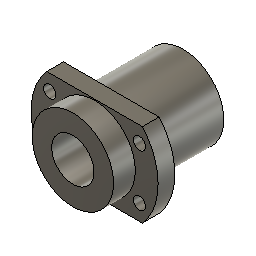
Prototype_1_reducer v30 (Autodesk Fusion 360 archive; units mm, degrees)
design "SFY4040-3.6"
Autodesk Fusion 360 part; units mm, degrees
sketch "Sketch1" plane through (0, 0, 0) normal (0, 0, 1) x (1, 0, 0)
  circle A0 centre (0, 0) radius 19
  circle A1 centre (0, 0) radius 57
  circle A2 centre (0, 0) radius 46.5 construction
  line L0 (57, 37.5) -> (-57, 37.5)
  line L1 (-57, 37.5) -> (-57, -37.5)
  line L2 (-57, -37.5) -> (57, -37.5)
  line L3 (57, -37.5) -> (57, 37.5)
  line L4 (57, 37.5) -> (-57, -37.5) construction
  line L5 (-57, 37.5) -> (57, -37.5) construction
  circle A3 centre (0, 0) radius 36.5
  dimension "d1" = 38
  dimension "d2" = 114
  dimension "d3" = 93
  dimension "d4" = 75
  dimension "d5" = 114
  dimension "d6" = 73
  constraint coincident A0.centre A1.centre
  constraint concentric A1 A2
  constraint perpendicular L0 L1
  constraint parallel L0 L2
  constraint parallel L1 L3
  constraint horizontal L0
  constraint coincident L4 A0.centre
  constraint coincident L5 A0.centre
  constraint concentric A2 A3
  measures "d1" diameter of A0
  measures "d2" diameter of A1
  measures "d3" diameter of A2
  measures "d4" distance of L0.start L2.end
  measures "d5" distance of L0.start L0.end
  measures "d6" diameter of A3
extrude "Extrude1" add sketch "Sketch1" against normal blind 15 contours A1 L0 L2 | A3
extrude "Extrude2" add sketch "Sketch1" along normal blind 19.5 contours A3
sketch "Sketch2" plane through (0, 0, -15) normal (0, 0, -1) x (-1, 0, 0)
  circle A0 centre (0, 0) radius 19
  arc A1 (42.9273, -37.5) -> (42.9273, 37.5) centre (0, 0) ccw
  line L0 (42.9273, 37.5) -> (-42.9273, 37.5)
  arc A2 (-42.9273, 37.5) -> (-42.9273, -37.5) centre (0, 0) ccw
  line L1 (-42.9273, -37.5) -> (42.9273, -37.5)
  circle A3 centre (0, 0) radius 36.5
  circle A4 centre (0, 0) radius 36.5
extrude "Extrude3" add sketch "Sketch2" along normal blind 64.5 contours A3 A4
sketch "Sketch3" plane through (0, 0, 0) normal (0, 0, 1) x (1, 0, 0)
  circle A0 centre (0, 0) radius 36.5
  arc A1 (-42.9273, 37.5) -> (-42.9273, -37.5) centre (0, 0) ccw
  line L0 (-42.9273, -37.5) -> (42.9273, -37.5)
  arc A2 (42.9273, -37.5) -> (42.9273, 37.5) centre (0, 0) ccw
  line L1 (42.9273, 37.5) -> (-42.9273, 37.5)
  circle A3 centre (0, 0) radius 46.5 construction
  line L2 (-57, -37.5) -> (57, -37.5)
  line L3 (57, -37.5) -> (57, 37.5)
  line L4 (-57, 37.5) -> (-57, -37.5)
  line L5 (57, 37.5) -> (-57, 37.5)
  line L6 (0, 0) -> (57, 0) construction
  circle A4 centre (40.2702, 23.25) radius 5.5
  line L7 (0, 0) -> (40.2702, 23.25)
  line L8 (0, 0) -> (0, 36.5) construction
  circle A5 centre (40.2702, -23.25) radius 5.5
  circle A6 centre (-40.2702, -23.25) radius 5.5
  circle A7 centre (-40.2702, 23.25) radius 5.5
  dimension "d13" = 11
  dimension "d14" = 30
  constraint coincident A0.centre A1.centre
  constraint midpoint L3 L6.end
  constraint coincident A3 A4.centre
  constraint coincident A4.centre L7.end
  constraint coincident A0 L8.end
  constraint perpendicular L6 L8
  constraint symmetric L6 A4 A5
  constraint symmetric A4 L8 A7
  constraint symmetric L8 A5 A6
  measures "d13" diameter of A4
  measures "d14" angle of L6 L7
extrude "Extrude4" cut sketch "Sketch3" against normal blind 16.266 contours A4 | A5 | A6 | A7

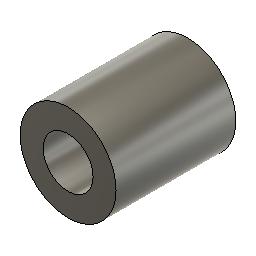
design "RCL48-2525"
Autodesk Fusion 360 part; units mm, degrees
sketch "Sketch1" plane through (0, 0, 0) normal (0, 0, 1) x (1, 0, 0)
  circle A0 centre (0, 0) radius 24
  dimension "d1" = 48
  constraint coincident A0.centre origin
  measures "d1" diameter of A0
extrude "Extrude1" add sketch "Sketch1" against normal blind 60
sketch "Sketch2" plane through (0, 0, 0) normal (0, 0, 1) x (1, 0, 0)
  circle A0 centre (0, 0) radius 24
  circle A1 centre (0, 0) radius 12.5
  dimension "d4" = 25
  constraint concentric A0 A1
  measures "d4" diameter of A1
extrude "Extrude2" cut sketch "Sketch2" against normal blind 84.022 contours A1

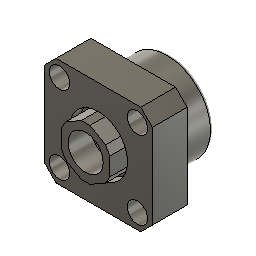
design "FK30"
Autodesk Fusion 360 part; units mm, degrees
sketch "Sketch1" plane through (0, 0, 0) normal (0, 0, 1) x (1, 0, 0)
  line L0 (46.5, 46.5) -> (-46.5, 46.5)
  line L1 (-46.5, 46.5) -> (-46.5, -46.5)
  line L2 (-46.5, -46.5) -> (46.5, -46.5)
  line L3 (46.5, -46.5) -> (46.5, 46.5)
  line L4 (46.5, 46.5) -> (-46.5, -46.5) construction
  line L5 (-46.5, 46.5) -> (46.5, -46.5) construction
  dimension "d1" = 93
  dimension "d2" = 93
  constraint perpendicular L0 L1
  constraint parallel L0 L2
  constraint parallel L1 L3
  constraint horizontal L0
  constraint coincident L4 origin
  constraint coincident L5 origin
  measures "d1" distance of L0.start L0.end
  measures "d2" distance of L0.start L2.end
extrude "Extrude1" add sketch "Sketch1" against normal blind 30 makes body 1
sketch "Sketch2" plane through (0, 0, -30) normal (0, 0, -1) x (-1, 0, 0)
  line L0 (-46.5, 46.5) -> (-46.5, -46.5)
  line L1 (-46.5, -46.5) -> (46.5, -46.5)
  line L2 (46.5, -46.5) -> (46.5, 46.5)
  line L3 (46.5, 46.5) -> (-46.5, 46.5)
  circle A0 centre (0, 0) radius 37.5
  dimension "d5" = 75
  constraint coincident A0.centre origin
  measures "d5" diameter of A0
extrude "Extrude2" add sketch "Sketch2" along normal blind 32 contours A0 bodies 1
sketch "Sketch3" plane through (0, 0, 0) normal (0, 0, 1) x (1, 0, 0)
  line L0 (46.5, -46.5) -> (46.5, 46.5)
  line L1 (46.5, 46.5) -> (-46.5, 46.5)
  line L2 (-46.5, 46.5) -> (-46.5, -46.5)
  line L3 (-46.5, -46.5) -> (46.5, -46.5)
  circle A0 centre (0, 0) radius 47.5 construction
  circle A1 centre (33.5876, 33.5876) radius 5.5
  circle A2 centre (33.5876, -33.5876) radius 5.5
  circle A3 centre (-33.5876, -33.5876) radius 5.5
  circle A4 centre (-33.5876, 33.5876) radius 5.5
  line L4 (0, 0) -> (46.5, 0) construction
  line L5 (33.5876, 33.5876) -> (0, 0) construction
  dimension "d8" = 95
  dimension "d9" = 11
  dimension "d10" = 45
  constraint coincident A0.centre L4.start
  constraint coincident A0 A1.centre
  constraint coincident A0 A2.centre
  constraint coincident A0 A3.centre
  constraint coincident A0 A4.centre
  constraint equal A1 A4
  constraint equal A3 A4
  constraint equal A2 A3
  constraint midpoint L0 L4.end
  constraint coincident A1.centre L5.start
  constraint horizontal A4.centre A1.centre
  constraint vertical A3.centre A4.centre
  constraint horizontal A2.centre A3.centre
  measures "d8" diameter of A0
  measures "d9" diameter of A1
  measures "d10" angle of L4 L5
extrude "Extrude3" cut sketch "Sketch3" against normal blind 34.907 contours A1 | A2 | A3 | A4 bodies 1
sketch "Sketch4" plane through (0, 0, 0) normal (0, 0, 1) x (1, 0, 0)
  circle A0 centre (-33.5876, 33.5876) radius 5.5
  circle A1 centre (-33.5876, -33.5876) radius 5.5
  circle A2 centre (33.5876, 33.5876) radius 5.5
  circle A3 centre (33.5876, -33.5876) radius 5.5
  line L0 (46.5, -46.5) -> (46.5, 46.5)
  line L1 (46.5, 46.5) -> (-46.5, 46.5)
  line L2 (-46.5, 46.5) -> (-46.5, -46.5)
  line L3 (-46.5, -46.5) -> (46.5, -46.5)
  circle A4 centre (33.5876, 33.5876) radius 8.75
  circle A5 centre (-33.5876, 33.5876) radius 8.75
  circle A6 centre (-33.5876, -33.5876) radius 8.75
  circle A7 centre (33.5876, -33.5876) radius 8.75
  dimension "d13" = 17.5
  constraint concentric A2 A4
  constraint concentric A0 A5
  constraint concentric A1 A6
  constraint concentric A3 A7
  constraint equal A4 A5
  constraint equal A5 A6
  constraint equal A6 A7
  measures "d13" diameter of A4
extrude "Extrude4" cut sketch "Sketch4" against normal blind 15 contours A4 | A5 | A6 | A7 bodies 1
sketch "Sketch5" plane through (0, 0, 0) normal (0, 0, 1) x (1, 0, 0)
  circle A0 centre (-33.5876, 33.5876) radius 8.75
  circle A1 centre (-33.5876, -33.5876) radius 8.75
  circle A2 centre (33.5876, 33.5876) radius 8.75
  circle A3 centre (33.5876, -33.5876) radius 8.75
  line L0 (46.5, -46.5) -> (46.5, 46.5)
  line L1 (46.5, 46.5) -> (-46.5, 46.5)
  line L2 (-46.5, 46.5) -> (-46.5, -46.5)
  line L3 (-46.5, -46.5) -> (46.5, -46.5)
  circle A4 centre (0, 0) radius 15
  dimension "d16" = 30
  constraint coincident A4.centre origin
  measures "d16" diameter of A4
extrude "Extrude5" cut sketch "Sketch5" against normal blind 68.719 contours A4 bodies 1
sketch "Sketch6" plane through (0, 0, 0) normal (0, 0, 1) x (1, 0, 0)
  circle A0 centre (0, 0) radius 15
  circle A1 centre (-33.5876, 33.5876) radius 8.75
  circle A2 centre (-33.5876, -33.5876) radius 8.75
  circle A3 centre (33.5876, 33.5876) radius 8.75
  circle A4 centre (33.5876, -33.5876) radius 8.75
  line L0 (46.5, -46.5) -> (46.5, 46.5)
  line L1 (46.5, 46.5) -> (-46.5, 46.5)
  line L2 (-46.5, 46.5) -> (-46.5, -46.5)
  line L3 (-46.5, -46.5) -> (46.5, -46.5)
  circle A5 centre (0, 0) radius 25
  dimension "d19" = 50
  constraint concentric A0 A5
  measures "d19" diameter of A5
extrude "Extrude6" cut sketch "Sketch6" against normal blind 9 contours A5 bodies 1
sketch "Sketch7" plane through (0, 0, -9) normal (0, 0, 1) x (1, 0, 0)
  circle A0 centre (0, 0) radius 15
  circle A1 centre (0, 0) radius 25
  circle A2 centre (0, 0) radius 22.5
  dimension "d22" = 45
  constraint concentric A0 A2
  measures "d22" diameter of A2
extrude "Extrude7" cut sketch "Sketch7" against normal blind 9 contours A2 bodies 1
sketch "Sketch8" plane through (0, 0, -18) normal (0, 0, 1) x (1, 0, 0)
  circle A0 centre (0, 0) radius 15
  circle A1 centre (0, 0) radius 22.5
  circle A2 centre (0, 0) radius 17.4
  dimension "d25" = 34.8
  constraint concentric A0 A2
  measures "d25" diameter of A2
extrude "Extrude8" add sketch "Sketch8" along normal blind 9 separate body contours A2 makes body 2
sketch "Sketch9" plane through (0, 0, -62) normal (0, 0, -1) x (-1, 0, 0)
  circle A0 centre (0, 0) radius 15
  circle A1 centre (0, 0) radius 37.5
  circle A2 centre (0, 0) radius 22.5
  dimension "d28" = 45
  constraint concentric A0 A2
  measures "d28" diameter of A2
extrude "Extrude9" cut sketch "Sketch9" against normal blind 12 contours A2 bodies 1
sketch "Sketch10" plane through (0, 0, -50) normal (0, 0, -1) x (-1, 0, 0)
  circle A0 centre (0, 0) radius 15
  circle A1 centre (0, 0) radius 22.5
  circle A2 centre (0, 0) radius 17.4
  dimension "d31" = 34.8
  constraint coincident A0.centre A1.centre
  measures "d31" diameter of A2
extrude "Extrude10" add sketch "Sketch10" along normal blind 9 separate body contours A2 makes body 3
chamfer "Chamfer1" distance 10 angle 45 4 edges at (46.5, 46.5, -15) (-46.5, 46.5, -15) (46.5, -46.5, -15) (-46.5, -46.5, -15) on bodies 1
fillet "Fillet1" radius 3 1 edges at (34.9623, -13.5606, -62) on bodies 1
sketch "Sketch11" plane through (0, 0, -9) normal (0, 0, 1) x (1, 0, 0)
  circle A0 centre (0, 0) radius 15
  circle A1 centre (0, 0) radius 17.4
  line L0 (0, 31.1127) -> (0, -31.1127) construction
  line L1 (-12.7017, 22) -> (-25.4034, 0)
  line L2 (-25.4034, 0) -> (-12.7017, -22)
  line L3 (-12.7017, -22) -> (12.7017, -22)
  line L4 (12.7017, -22) -> (25.4034, 0)
  line L5 (25.4034, 0) -> (12.7017, 22)
  line L6 (12.7017, 22) -> (-12.7017, 22)
  dimension "d43" = 22
  constraint coincident A0.centre A1.centre
  constraint coincident L0 A0.centre
  constraint vertical L0
  constraint horizontal L6
  measures "d43" distance of A0.centre L6
extrude "Extrude11" add sketch "Sketch11" along normal blind 20 separate body contours A1 | L1 L2 L3 L4 L5 L6 makes body 4
chamfer "Chamfer4" distance 9 angle 45 6 edges at (12.7017, 22, 1) (25.4034, 0, 1) (12.7017, -22, 1) (-12.7017, -22, 1) (-25.4034, 0, 1) (-12.7017, 22, 1) on bodies 4

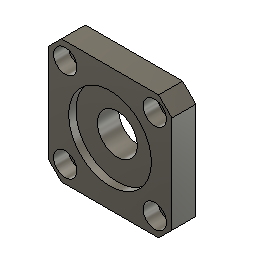
design "FF30"
Autodesk Fusion 360 part; units mm, degrees
sketch "Sketch1" plane through (0, 0, 0) normal (0, 0, 1) x (1, 0, 0)
  line L0 (46.5, 46.5) -> (-46.5, 46.5)
  line L1 (-46.5, 46.5) -> (-46.5, -46.5)
  line L2 (-46.5, -46.5) -> (46.5, -46.5)
  line L3 (46.5, -46.5) -> (46.5, 46.5)
  line L4 (46.5, 46.5) -> (-46.5, -46.5) construction
  line L5 (-46.5, 46.5) -> (46.5, -46.5) construction
  dimension "d1" = 93
  dimension "d2" = 93
  constraint perpendicular L0 L1
  constraint parallel L0 L2
  constraint parallel L1 L3
  constraint horizontal L0
  constraint coincident L4 origin
  constraint coincident L5 origin
  measures "d1" distance of L0.start L0.end
  measures "d2" distance of L0.start L2.end
extrude "Extrude1" add sketch "Sketch1" against normal blind 18
sketch "Sketch2" plane through (0, 0, -18) normal (0, 0, -1) x (-1, 0, 0)
  line L0 (-46.5, 46.5) -> (-46.5, -46.5)
  line L1 (-46.5, -46.5) -> (46.5, -46.5)
  line L2 (46.5, -46.5) -> (46.5, 46.5)
  line L3 (46.5, 46.5) -> (-46.5, 46.5)
  circle A0 centre (0, 0) radius 37.5
  dimension "d5" = 75
  constraint coincident A0.centre origin
  measures "d5" diameter of A0
extrude "Extrude2" add sketch "Sketch2" along normal blind 9 contours A0
sketch "Sketch3" plane through (0, 0, 0) normal (0, 0, 1) x (1, 0, 0)
  line L0 (46.5, -46.5) -> (46.5, 46.5)
  line L1 (46.5, 46.5) -> (-46.5, 46.5)
  line L2 (-46.5, 46.5) -> (-46.5, -46.5)
  line L3 (-46.5, -46.5) -> (46.5, -46.5)
  circle A0 centre (0, 0) radius 15
  dimension "d8" = 30
  constraint coincident A0.centre origin
  measures "d8" diameter of A0
extrude "Extrude3" cut sketch "Sketch3" against normal blind 60.226 contours A0
sketch "Sketch4" plane through (0, 0, 0) normal (0, 0, 1) x (1, 0, 0)
  circle A0 centre (0, 0) radius 15
  line L0 (46.5, -46.5) -> (46.5, 46.5)
  line L1 (46.5, 46.5) -> (-46.5, 46.5)
  line L2 (-46.5, 46.5) -> (-46.5, -46.5)
  line L3 (-46.5, -46.5) -> (46.5, -46.5)
  circle A1 centre (0, 0) radius 31
  dimension "d11" = 62
  constraint concentric A0 A1
  measures "d11" diameter of A1
extrude "Extrude4" cut sketch "Sketch4" against normal blind 5.5 contours A1
sketch "Sketch5" plane through (0, 0, -27) normal (0, 0, -1) x (-1, 0, 0)
  circle A0 centre (0, 0) radius 15
  circle A1 centre (0, 0) radius 37.5
  circle A2 centre (0, 0) radius 31
  dimension "d14" = 62
  constraint concentric A0 A2
  measures "d14" diameter of A2
extrude "Extrude5" cut sketch "Sketch5" against normal blind 5.5 contours A2
chamfer "Chamfer1" distance 10 angle 45 4 edges at (46.5, 46.5, -9) (-46.5, 46.5, -9) (-46.5, -46.5, -9) (46.5, -46.5, -9)
sketch "Sketch6" plane through (0, 0, 0) normal (0, 0, 1) x (1, 0, 0)
  line L0 (36.5, -46.5) -> (46.5, -36.5)
  line L1 (46.5, -36.5) -> (46.5, 36.5)
  line L2 (46.5, 36.5) -> (36.5, 46.5)
  line L3 (36.5, 46.5) -> (-36.5, 46.5)
  line L4 (-36.5, 46.5) -> (-46.5, 36.5)
  line L5 (-46.5, 36.5) -> (-46.5, -36.5)
  line L6 (-46.5, -36.5) -> (-36.5, -46.5)
  line L7 (-36.5, -46.5) -> (36.5, -46.5)
  circle A0 centre (0, 0) radius 31
  circle A1 centre (0, 0) radius 47.5 construction
  circle A2 centre (33.5876, 33.5876) radius 5.5
  circle A3 centre (-33.5876, 33.5876) radius 5.5
  circle A4 centre (-33.5876, -33.5876) radius 5.5
  circle A5 centre (33.5876, -33.5876) radius 5.5
  line L8 (0, 0) -> (46.5, 0) construction
  line L9 (33.5876, 33.5876) -> (0, 0) construction
  dimension "d18" = 95
  dimension "d19" = 11
  dimension "d20" = 45
  constraint concentric A0 A1
  constraint coincident A1 A2.centre
  constraint coincident A1 A3.centre
  constraint coincident A1 A4.centre
  constraint coincident A1 A5.centre
  constraint equal A2 A3
  constraint equal A3 A4
  constraint equal A4 A5
  constraint coincident A0.centre A1.centre
  constraint midpoint L1 L8.end
  constraint coincident A2.centre L9.start
  constraint horizontal A3.centre A2.centre
  constraint vertical A3.centre A4.centre
  constraint horizontal A4.centre A5.centre
  measures "d18" diameter of A1
  measures "d19" diameter of A2
  measures "d20" angle of L8 L9
extrude "Extrude6" cut sketch "Sketch6" against normal blind 23.985 contours A2 | A3 | A4 | A5
sketch "Sketch7" plane through (0, 0, 0) normal (0, 0, 1) x (1, 0, 0)
  circle A0 centre (33.5876, 33.5876) radius 5.5
  circle A1 centre (33.5876, -33.5876) radius 5.5
  circle A2 centre (-33.5876, 33.5876) radius 5.5
  circle A3 centre (-33.5876, -33.5876) radius 5.5
  line L0 (36.5, -46.5) -> (46.5, -36.5)
  line L1 (46.5, -36.5) -> (46.5, 36.5)
  line L2 (46.5, 36.5) -> (36.5, 46.5)
  line L3 (36.5, 46.5) -> (-36.5, 46.5)
  line L4 (-36.5, 46.5) -> (-46.5, 36.5)
  line L5 (-46.5, 36.5) -> (-46.5, -36.5)
  line L6 (-46.5, -36.5) -> (-36.5, -46.5)
  line L7 (-36.5, -46.5) -> (36.5, -46.5)
  circle A4 centre (0, 0) radius 31
  circle A5 centre (33.5876, 33.5876) radius 8.75
  circle A6 centre (-33.5876, 33.5876) radius 8.75
  circle A7 centre (-33.5876, -33.5876) radius 8.75
  circle A8 centre (33.5876, -33.5876) radius 8.75
  dimension "d23" = 17.5
  constraint concentric A0 A5
  constraint concentric A2 A6
  constraint concentric A3 A7
  constraint concentric A1 A8
  constraint equal A5 A6
  constraint equal A6 A7
  constraint equal A7 A8
  measures "d23" diameter of A5
extrude "Extrude7" cut sketch "Sketch7" against normal blind 11 contours A5 | A6 | A7 | A8

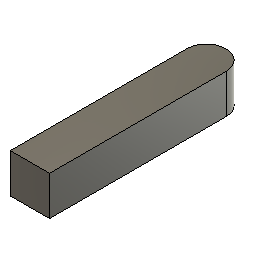
design "KEGH6-30"
Autodesk Fusion 360 part; units mm, degrees
sketch "Sketch1" plane through (0, 0, 0) normal (0, 1, 0) x (1, 0, 0)
  line L0 (3, 15) -> (-3, 15)
  line L1 (-3, 15) -> (-3, -15)
  line L2 (-3, -15) -> (3, -15)
  line L3 (3, -15) -> (3, 15)
  line L4 (3, 15) -> (-3, -15) construction
  line L5 (-3, 15) -> (3, -15) construction
  dimension "d1" = 30
  dimension "d2" = 6
  constraint perpendicular L0 L1
  constraint parallel L0 L2
  constraint parallel L1 L3
  constraint horizontal L0
  constraint coincident L4 origin
  constraint coincident L5 origin
  measures "d1" distance of L0.start L2.end
  measures "d2" distance of L1.end L2.end
extrude "Extrude1" add sketch "Sketch1" along normal blind 6
fillet "Fillet1" radius 3 2 edges at (3, 3, -15) (-3, 3, -15)

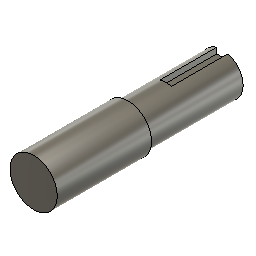
design "HandleShaft"
Autodesk Fusion 360 part; units mm, degrees
sketch "Sketch1" plane through (0, 0, 0) normal (0, 0, 1) x (1, 0, 0)
  circle A0 centre (0, 0) radius 12.5
  dimension "d1" = 25
  constraint coincident A0.centre origin
  measures "d1" diameter of A0
extrude "Extrude1" add sketch "Sketch1" against normal blind 50
sketch "Sketch2" plane through (0, 0, -50) normal (0, 0, -1) x (-1, 0, 0)
  circle A0 centre (0, 0) radius 12.5
  circle A1 centre (0, 0) radius 11
  dimension "d4" = 22
  constraint concentric A0 A1
  measures "d4" diameter of A1
extrude "Extrude2" add sketch "Sketch2" along normal blind 50 contours A1
sketch "Sketch3" plane through (0, 0, -100) normal (0, 0, -1) x (-1, 0, 0)
  circle A0 centre (0, 0) radius 11
  line L0 (-10.5014, 11) -> (10.5014, 11)
  line L1 (0, 0) -> (0, 11)
  line L2 (3, 11) -> (-3, 11)
  line L3 (-3, 11) -> (-3, 7.5)
  line L4 (-3, 7.5) -> (3, 7.5)
  line L5 (3, 7.5) -> (3, 11)
  point P0 (0, 7.5)
  dimension "d7" = 6
  dimension "d8" = 3.5
  constraint horizontal L0
  constraint tangent A0 L0
  constraint coincident A0.centre L1.start
  constraint midpoint L0 L1.end
  constraint vertical L1
  constraint horizontal L2
  constraint vertical L3
  constraint horizontal L4
  constraint vertical L5
  constraint coincident L0 L2.start
  constraint midpoint L4 P0
  constraint coincident L1 P0
  measures "d7" distance of L3.end L4.end
  measures "d8" distance of L2.start L4.end
extrude "Extrude3" cut sketch "Sketch3" against normal blind 30 contours A0 L1 L4 L5 | A0 L1 L3 L4
